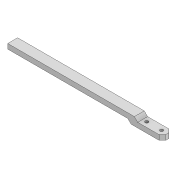
# Autodesk Inventor part: spazzola - asta
Saved by Autodesk Inventor 2022 (Build 260153000, 153)
## iProperties
Created: 2025-08-09
Part Number: spazzola - asta
Material: Generic
Document SubType Name: Modeling
Designer: sacchie
Density: 1 g/cm^3
Appearance: Default
Author: sacchie
Autodesk Inventor part; units mm, degrees
ref_plane "YZ Plane" through (0, 0, 0) normal (1, 0, 0) x (0, 1, 0)
ref_plane "XZ Plane" through (0, 0, 0) normal (0, 1, 0) x (-1, 0, 0)
ref_plane "XY Plane" through (0, 0, 0) normal (0, 0, 1) x (1, 0, 0)
sketch "Sketch1" plane through (0, 0, 0) normal (0, 0, 1) x (1, 0, 0)
  line L0 (0, 0) -> (-19, 0)
  line L1 (-19, 0) -> (-19, 2)
  line L2 (-19, 2) -> (-94, 2)
  line L3 (-94, 2) -> (-94, 5)
  line L4 (-94, 5) -> (-17, 5)
  line L5 (-17, 5) -> (-17, 3)
  line L6 (-17, 3) -> (0, 3)
  line L7 (0, 3) -> (0, 0)
  dimension "d1" = 2
  dimension "d3" = 3
  dimension "d4" = 3
  dimension "d5" = 17
  dimension "d6" = 2
  dimension "d7" = 75
  constraints: 16 end point, 6 perpendicular, 1 horizontal, 1 vertical
  measures "d1" distance of L4.end L5.end
  measures "d3" distance between parallel lines of L4 L2
  measures "d4" distance between parallel lines of L6 L0
  measures "d5" distance between parallel lines of L7 L5
  measures "d6" distance between parallel lines of L5 L1
  measures "d7" distance of L1.end L2.end
extrude "Extrusion1" add sketch "Sketch1" along normal blind 6
chamfer "Chamfer1" distance 2 angle 45 2 edges at (0, 1.5, 0) (0, 1.5, 6)
sketch "Sketch2" plane through (-17, 3, 6) normal (0, 1, 0) x (1, 0, 0)
  line L0 (0, 6) -> (0, 0) projected
  line L1 (0, 3) -> (27, 3) construction
  circle A0 centre (13.5, 3) radius 1
  circle A1 centre (4.5, 3) radius 1
  line L2 (17, 4) -> (17, 2) projected
  point P0 (17, 6)
  dimension "d13" = 2
  dimension "d14" = 2
  dimension "d15" = 9
  dimension "d16" = 3.5
  constraints: 2 centre point, 2 end point, 2 midpoint, 1 horizontal, 1 point on line
  measures "d13" diameter of A0
  measures "d14" diameter of A1
  measures "d15" distance of A0.centre A1.centre
  measures "d16" distance from line of L2 A0.centre
extrude "Extrusion2" cut sketch "Sketch2" against normal through all
sketch "Sketch3" plane through (-94, 2, 0) normal (-1, 0, 0) x (0, 0, 1)
  line L0 (3, 0) -> (3, 4.5868) construction
  line L1 (0.8, 1.5) -> (1.5, 0)
  line L2 (1.5, 0) -> (4.5, 0)
  line L3 (4.5, 0) -> (5.2, 1.5)
  line L4 (5.2, 1.5) -> (0.8, 1.5)
  line L5 (0, 0) -> (6, 0) projected
  point P0 (0, -2)
  dimension "d20" = 1.5
  dimension "d21" = 2.2
  dimension "d22" = 4.4
  dimension "d23" = 3
  dimension "d24" = 1.5
  constraints: 10 end point, 1 collinear, 1 vertical
  measures "d20" distance from line of L0 L1.end
  measures "d21" distance from line of L1.start L0
  measures "d22" distance of L3.end L1.start
  measures "d23" distance of L2.end L1.end
  measures "d24" distance between parallel lines of L2 L4
extrude "Extrusion3" cut sketch "Sketch3" against normal blind 72
chamfer "Chamfer2" distance 2 angle 45 1 edges at (-19, 2, 3)
chamfer "Chamfer3" distance 2 distance2 2 1 edges at (-17, 3, 3) measured on face at (-16.5, 3, 3)
equation "\"d14\" = d13"
equation "\"d20\" = 0.5 * d23"
equation "\"d21\" = 0.5 * d22"
body "Solid1"
